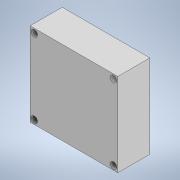
# Autodesk Inventor part: imx291CameraModule
Saved by Autodesk Inventor 2022.1 (Build 261234000, 234)
## iProperties
Created: 2021-07-20
Part Number: imx291CameraModule
Material: Generic
Document SubType Name: Modeling
Designer: robst
Density: 1 g/cm^3
Appearance: Default
Author: robst
Autodesk Inventor part; units mm, degrees
ref_plane "YZ Plane" through (0, 0, 0) normal (1, 0, 0) x (0, 1, 0)
ref_plane "XZ Plane" through (0, 0, 0) normal (0, 1, 0) x (-1, 0, 0)
ref_plane "XY Plane" through (0, 0, 0) normal (0, 0, 1) x (1, 0, 0)
sketch "Sketch1" plane through (0, 0, 0) normal (0, 0, 1) x (1, 0, 0)
  line L0 (-20.5, -19.5) -> (20.5, -19.5)
  line L1 (20.5, -19.5) -> (20.5, 19.5)
  line L2 (20.5, 19.5) -> (-20.5, 19.5)
  line L3 (-20.5, 19.5) -> (-20.5, -19.5)
  line L4 (-20.5, -19.5) -> (20.5, 19.5) construction
  line L5 (20.5, -19.5) -> (-20.5, 19.5) construction
  line L6 (-18.5, -17.5) -> (18.5, -17.5) construction
  line L7 (18.5, -17.5) -> (18.5, 17.5) construction
  line L8 (18.5, 17.5) -> (-18.5, 17.5) construction
  line L9 (-18.5, 17.5) -> (-18.5, -17.5) construction
  line L10 (-18.5, -17.5) -> (18.5, 17.5) construction
  line L11 (18.5, -17.5) -> (-18.5, 17.5) construction
  circle A0 centre (-18.5, 17.5) radius 1.5
  circle A1 centre (18.5, 17.5) radius 1.5
  circle A2 centre (18.5, -17.5) radius 1.5
  circle A3 centre (-18.5, -17.5) radius 1.5
  point P0 (0, 0)
  dimension "d0" = 41
  dimension "d1" = 39
  dimension "d2" = 37
  dimension "d3" = 35
  dimension "d4" = 3
  constraints: 24 end point, 5 coincident, 4 centre point, 4 midpoint, 4 parallel, 3 equal radius, 2 horizontal, 2 perpendicular
  measures "d0" distance of L1.end L2.end
  measures "d1" distance of L2.end L0.start
  measures "d2" distance of L7.end L8.end
  measures "d3" distance of L8.end L6.start
  measures "d4" diameter of A0
extrude "Extrusion1" add sketch "Sketch1" against normal blind 15
equation "\"d0\" = imx291ModuleWidth"
equation "\"d1\" = imx291ModuleLength"
equation "\"d2\" = imx291ModuleScrewWidthDistance"
equation "\"d3\" = imx291ModuleScrewLengthDistance"
equation "\"d4\" = screwDiameterHole"
equation "\"d5\" = imx291ModuleDepth"
equation "\"imx291ModuleWidth\" = 41"
equation "\"imx291ModuleLength\" = 39"
equation "\"imx291ModuleDepth\" = 15"
equation "\"imx291ModuleScrewWidthDistance\" = 37"
equation "\"imx291ModuleScrewLengthDistance\" = 35"
equation "\"screwDiameterHole\" = 3"
body "Solid1"
